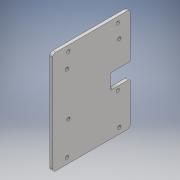
# Autodesk Inventor part: adapter_arduino_to_power
Saved by Autodesk Inventor 2018 (Build 220112000, 112)
## iProperties
Created: 2019-05-08
Part Number: adapter_arduino_to_power
Material: Типовые
Document SubType Name: Modeling
Designer: KV33_HP1
Density: 1 g/cm^3
Appearance: По умолчанию
Author: KV33_HP1
Autodesk Inventor part; units mm, degrees
ref_plane "YZ Plane" through (0, 0, 0) normal (1, 0, 0) x (0, 1, 0)
ref_plane "XZ Plane" through (0, 0, 0) normal (0, 1, 0) x (-1, 0, 0)
ref_plane "XY Plane" through (0, 0, 0) normal (0, 0, 1) x (1, 0, 0)
sketch "Эскиз1" plane through (0, 0, 0) normal (1, 0, 0) x (0, 1, 0)
  circle A0 centre (0, 0) radius 1.65
  circle A1 centre (0, -76) radius 1.65
  circle A2 centre (-52, 0) radius 1.65
  circle A3 centre (-52, -76) radius 1.65
  line L0 (-63, 20) -> (8, 20)
  line L1 (8, -82) -> (-63, -82)
  line L2 (-66, -79) -> (-66, 17)
  arc A4 (11, 17) -> (8, 20) centre (8, 17) ccw
  arc A5 (8, -82) -> (11, -79) centre (8, -79) ccw
  arc A6 (-66, -79) -> (-63, -82) centre (-63, -79) ccw
  arc A7 (-63, 20) -> (-66, 17) centre (-63, 17) ccw
  circle A8 centre (-1.5, -43.6662) radius 1.65
  circle A9 centre (-50.5, -43.6662) radius 1.65
  circle A10 centre (-1.5, 14.3338) radius 1.65
  circle A11 centre (-50.5, 14.3338) radius 1.65
  line L3 (9, -39.8501) -> (-7, -39.8501)
  line L4 (-9, -37.8501) -> (-9, -26.8501)
  line L5 (-7, -24.8501) -> (9, -24.8501)
  line L6 (11, 17) -> (11, -22.8501)
  line L7 (11, -41.8501) -> (11, -79)
  arc A12 (-9, -37.8501) -> (-7, -39.8501) centre (-7, -37.8501) ccw
  arc A13 (-7, -24.8501) -> (-9, -26.8501) centre (-7, -26.8501) ccw
  arc A14 (9, -24.8501) -> (11, -22.8501) centre (9, -22.8501) ccw
  arc A15 (11, -41.8501) -> (9, -39.8501) centre (9, -41.8501) ccw
  point P0 (11, -39.8501)
  point P1 (-9, -39.8501)
  point P2 (-9, -24.8501)
  dimension "d4" = 3.3
  dimension "d8" = 3.3
  dimension "d13" = 3.3
  dimension "d14" = 3.3
  dimension "d20" = 3
  dimension "d23" = 52
  dimension "d29" = 3.3
  dimension "d31" = 3.3
  dimension "d34" = 3.3
  dimension "d35" = 3.3
  dimension "d36" = 20
  dimension "d37" = 15
  dimension "d38" = 2
  constraints: 18 tangent, 16 centre point, 16 end point, 16 point on circle, 6 equal radius, 6 point on line, 5 perpendicular, 3 parallel, 2 horizontal, 1 coincident
  measures "d4" diameter of A0
  measures "d8" diameter of A1
  measures "d13" diameter of A2
  measures "d14" diameter of A3
  measures "d20" radius of A4
  measures "d23" distance of A3.centre A1.centre
  measures "d29" diameter of A8
  measures "d31" diameter of A9
  measures "d34" diameter of A10
  measures "d35" diameter of A11
  measures "d36" distance of point (11, -39.85) point (-9, -39.85)
  measures "d37" distance of point (-9, -39.85) point (-9, -24.85)
  measures "d38" radius of A12
extrude "Выдавливание2" add sketch "Эскиз1" along normal blind 3
